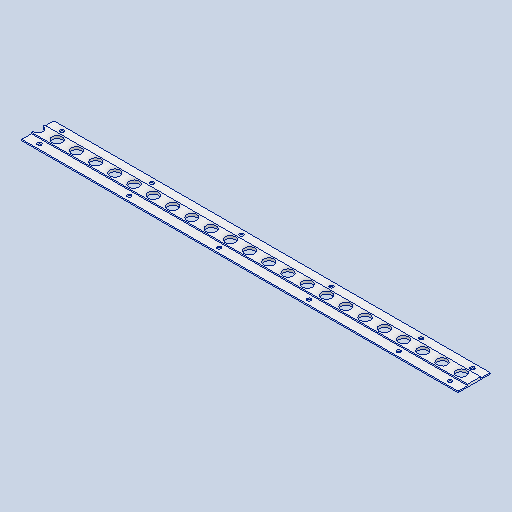
# Autodesk Inventor part: link1plate2
Saved by Autodesk Inventor 2024 (Build 280153000, 153)
## iProperties
Created: 2025-02-07
Part Number: link1plate2
Material: アルミニウム 6061
Document SubType Name: Modeling
Designer: tanoue_kota
Density: 2.7 g/cm^3
Appearance: アルミニウム - フラット
Mass: 25.7782 g
Surface Area: 172.187 cm^2
Volume: 9.54748 cm^3
Author: tanoue_kota
Autodesk Inventor part; units mm, degrees
ref_plane "YZ Plane" through (0, 0, 0) normal (1, 0, 0) x (0, 1, 0)
ref_plane "XZ Plane" through (0, 0, 0) normal (0, 1, 0) x (-1, 0, 0)
ref_plane "XY Plane" through (0, 0, 0) normal (0, 0, 1) x (1, 0, 0)
sketch "スケッチ1" plane through (0, 0, 0) normal (0, 1, 0) x (-1, 0, 0)
  line L0 (0, 0) -> (-340, 0)
  line L1 (-340, 0) -> (-340, -25)
  line L2 (-340, -25) -> (0, -25)
  line L3 (0, -25) -> (0, 0)
  dimension "d0" = 340
  dimension "d1" = 25
  constraints: 8 end point, 2 parallel, 1 horizontal, 1 perpendicular
  measures "d0" distance of L1.end L2.end
  measures "d1" distance of L0.end L1.end
extrude "押し出し1" add sketch "スケッチ1" along normal blind 2
sketch "スケッチ2" plane through (0, 2, 0) normal (0, 1, 0) x (1, 0, 0)
  line L0 (0, 25) -> (0, 0) projected
  line L1 (0, 12.5) -> (340, 12.5)
  line L2 (340, 0) -> (340, 25) projected
  line L3 (0, 12.5) -> (340, 12.5)
  line L4 (340, 12.5) -> (340, 17.5)
  line L5 (340, 17.5) -> (0, 17.5)
  line L6 (0, 17.5) -> (0, 12.5)
  line L7 (0, 0) -> (0, 25)
  line L8 (340, 25) -> (340, 0)
  line L9 (340, 7.5) -> (0, 7.5)
  line L10 (0, 0) -> (340, 0)
  line L11 (340, 0) -> (340, 25)
  line L12 (340, 25) -> (0, 25)
  line L13 (0, 25) -> (0, 0)
  point P0 (0, 17.5)
  point P1 (0, 7.5)
  dimension "d4" = 5
  constraints: 24 end point, 6 symmetric about line, 4 parallel, 2 horizontal, 2 midpoint, 2 perpendicular, 2 point on line
  measures "d4" distance between parallel lines of L1 L5
extrude "押し出し2" cut sketch "スケッチ2" against normal blind 1 contours L12 L2 L5 L0 | L9 L2 L10 L0
sketch "スケッチ3" plane through (0, 1, 0) normal (0, 1, 0) x (1, 0, 0)
  line L0 (0, 0) -> (0, 7.5) projected
  line L1 (0, 3.75) -> (340, 3.75)
  line L2 (340, 7.5) -> (340, 0) projected
  line L3 (340, 7.5) -> (340, 17.5) projected
  line L4 (340, 12.5) -> (0, 12.5)
  line L5 (0, 17.5) -> (0, 7.5) projected
  point P0 (10, 3.75)
  point P1 (80, 3.75)
  point P2 (150, 3.75)
  point P3 (220, 3.75)
  point P4 (290, 3.75)
  point P5 (10, 21.25)
  point P6 (80, 21.25)
  point P7 (150, 21.25)
  point P8 (220, 21.25)
  point P9 (290, 21.25)
  point P10 (330, 3.75)
  point P11 (330, 21.25)
  dimension "d7" = 10
  dimension "d8" = 70
  dimension "d11" = 70
  dimension "d38" = 10
  constraints: 6 symmetric about line, 4 end point, 4 midpoint, 3 point on line, 1 horizontal, 3 other
  measures "d7" distance from line of L0 point (10, 3.75)
  measures "d8" distance of point (10, 3.75) point (80, 3.75)
  measures "d11" distance of point (80, 3.75) point (150, 3.75)
  measures "d38" distance from line of L2 point (330, 3.75)
hole "穴1" at (10, 1, -3.75) at (80, 1, -3.75) at (150, 1, -3.75) at (220, 1, -3.75) at (290, 1, -3.75) at (10, 1, -21.25) at (80, 1, -21.25) at (150, 1, -21.25) at (220, 1, -21.25) at (290, 1, -21.25) at (330, 1, -21.25) at (330, 1, -3.75) direction (0, -1, 0) diameter 3.1 end through all
sketch "スケッチ4" plane through (0, 2, 0) normal (0, 1, 0) x (1, 0, 0)
  line L0 (340, 0) -> (340, 25) projected
  line L1 (340, 12.5) -> (0, 12.5)
  line L2 (0, 17.5) -> (0, 7.5) projected
  point P0 (0, 0)
  point P1 (330, 12.5)
  point P2 (315, 12.5)
  point P3 (300, 12.5)
  point P4 (285, 12.5)
  point P5 (270, 12.5)
  point P6 (255, 12.5)
  point P7 (240, 12.5)
  point P8 (225, 12.5)
  point P9 (210, 12.5)
  point P10 (195, 12.5)
  point P11 (180, 12.5)
  point P12 (165, 12.5)
  point P13 (150, 12.5)
  point P14 (135, 12.5)
  point P15 (120, 12.5)
  point P16 (105, 12.5)
  point P17 (90, 12.5)
  point P18 (75, 12.5)
  point P19 (60, 12.5)
  point P20 (45, 12.5)
  point P21 (30, 12.5)
  point P22 (15, 12.5)
  point P23 (0, 12.5)
  dimension "d23" = 10
  dimension "d26" = 15
  constraints: 2 end point, 2 midpoint, 1 horizontal, 1 point on line, 22 other
  measures "d23" distance from line of L0 point (330, 12.5)
  measures "d26" distance of point (330, 12.5) point (315, 12.5)
hole "穴2" at (330, 2, -12.5) at (315, 2, -12.5) at (300, 2, -12.5) at (285, 2, -12.5) at (270, 2, -12.5) at (255, 2, -12.5) at (240, 2, -12.5) at (225, 2, -12.5) at (210, 2, -12.5) at (195, 2, -12.5) at (180, 2, -12.5) at (165, 2, -12.5) at (150, 2, -12.5) at (135, 2, -12.5) at (120, 2, -12.5) at (105, 2, -12.5) at (90, 2, -12.5) at (75, 2, -12.5) at (60, 2, -12.5) at (45, 2, -12.5) at (30, 2, -12.5) at (15, 2, -12.5) at (0, 2, -12.5) direction (0, -1, 0) diameter 8 depth 8 tip angle 118
equation "\"d0\" = polygon_len1"
equation "\"d4\" = 0.5 * polygon_wid3"
equation "\"polygon_len1\" = 340"
equation "\"polygon_wid3\" = 10"
